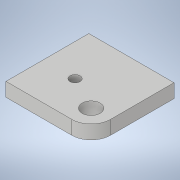
# Autodesk Inventor part: lw_6_part2
Saved by Autodesk Inventor 2021 (Build 250183000, 183)
## iProperties
Created: 2021-05-14
Part Number: lw_6_part2
Material: Типовые
Document SubType Name: Modeling
Designer: Kurbatova
Density: 1 g/cm^3
Appearance: По умолчанию
Author: Kurbatova
Autodesk Inventor part; units mm, degrees
ref_plane "YZ Plane" through (0, 0, 0) normal (1, 0, 0) x (0, 1, 0)
ref_plane "XZ Plane" through (0, 0, 0) normal (0, 1, 0) x (-1, 0, 0)
ref_plane "XY Plane" through (0, 0, 0) normal (0, 0, 1) x (1, 0, 0)
sketch "Эскиз1" plane through (0, 0, 0) normal (0, 0, 1) x (1, 0, 0)
  line L0 (-90.9717, -10.4774) -> (94.0283, -10.4774)
  line L1 (94.0283, -10.4774) -> (94.0283, 19.5226)
  line L2 (94.0283, 19.5226) -> (-90.9717, 19.5226)
  line L3 (-90.9717, 19.5226) -> (-90.9717, -10.4774)
  dimension "d2" = 185
  dimension "parametr_D" = 30
  constraints: 8 end point, 2 perpendicular, 1 horizontal, 1 vertical
  measures "d2" distance of L0.start L0.end
  measures "parametr_D" distance of L0.end L1.end
extrude "Выдавливание1" add sketch "Эскиз1" along normal blind 180
fillet "Сопряжение1" radius 42 1 edges at (94.0283, 4.5226, 180)
sketch "Эскиз7" plane through (-90.9717, 19.5226, 0) normal (0, 1, 0) x (1, 0, 0)
  point P0 (70, -100)
hole "Отверстие5" at (-20.9717, 19.5226, 100) direction (0, -1, 0) diameter 22 end through all
sketch "Эскиз8" plane through (-90.9717, 19.5226, 0) normal (0, 1, 0) x (1, 0, 0)
  point P0 (143, -138)
hole "Отверстие6" at (52.0283, 19.5226, 138) direction (0, -1, 0) diameter 39 end through all
sketch "Эскиз3" plane through (-90.9717, -10.4774, 0) normal (0, -1, 0) x (1, 0, 0)
  point P0 (115, 21.3555)
sketch "Эскиз4" plane through (-90.9717, -10.4774, 0) normal (0, -1, 0) x (1, 0, 0)
  point P0 (15, 33)
equation "\"d2\" = parametr_A_"
equation "\"parametr_D\" = parametr_C_"
equation "\"d4\" = parametr_B_"
equation "\"d26\" = parametr_G_"
equation "\"parametr_A_\" = 185"
equation "\"parametr_C_\" = 30"
equation "\"parametr_B_\" = 180"
equation "\"parametr_G_\" = 42"
